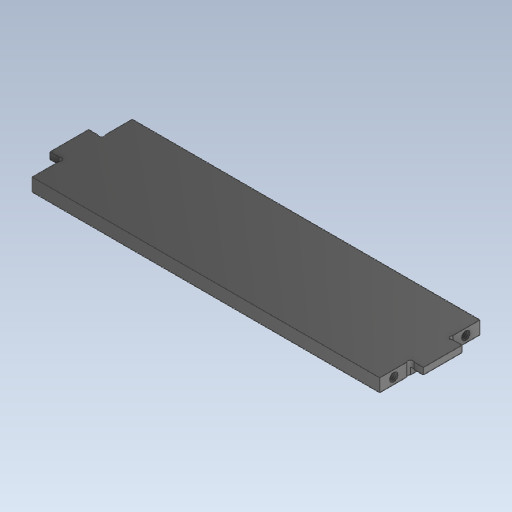
# Autodesk Inventor part: Cockpit_battery_bottom_frame
Saved by Autodesk Inventor 2020.4 (Build 244396000, 396)
## iProperties
Created: 2022-01-27
Part Number: Cockpit_battery_bottom_frame
Material: アセタール樹脂、黒
Document SubType Name: Modeling
Designer: Masato Kubotera
Density: 1.425 g/cm^3
Appearance: 滑らか - 黒
Author: Masato Kubotera
Autodesk Inventor part; units mm, degrees
ref_plane "YZ Plane" through (0, 0, 0) normal (1, 0, 0) x (0, 1, 0)
ref_plane "XZ Plane" through (0, 0, 0) normal (0, 1, 0) x (-1, 0, 0)
derived "Cockpit_side_frame_.ipt"
sketch "スケッチ2" plane through (0, 0, 0) normal (0, 1, 0) x (-1, 0, 0)
  line L0 (-28.5, -22.5) -> (86.5, -22.5) construction
  line L1 (86.5, -22.5) -> (86.5, -138.5)
  line L2 (86.5, -96) -> (-28.5, -96) construction
  line L3 (-28.5, -96) -> (-28.5, -22.5) construction
  line L4 (-28.5, -22.5) -> (86.5, -96) construction
  line L5 (86.5, -22.5) -> (-28.5, -96) construction
  line L6 (36.5, -101) -> (36.5, -133.5)
  line L7 (41.5, -138.5) -> (86.5, -138.5)
  arc A0 (62.6349, -70.4) -> (61.15, -71.8849) centre (61.8925, -71.1425) ccw
  arc A1 (71.15, -72.5349) -> (69.6651, -71.05) centre (70.4075, -71.7925) ccw
  line L8 (63.3349, -71.05) -> (69.6651, -71.05)
  line L9 (62.6349, -70.4) -> (70.3651, -70.4)
  line L10 (61.9, -71.1) -> (71.1, -71.1) construction
  arc A2 (63.3349, -71.05) -> (61.85, -72.5349) centre (62.5925, -71.7925) ccw
  line L11 (61.2, -70.45) -> (71.8, -70.45) construction
  line L12 (71.15, -72.5349) -> (71.15, -83.4651)
  line L13 (71.8, -78) -> (61.2, -78) construction
  line L14 (71.85, -71.8849) -> (71.85, -84.1151)
  line L15 (71.1, -71.1) -> (71.1, -84.9) construction
  line L16 (61.85, -72.5349) -> (61.85, -83.4651)
  line L17 (71.8, -70.45) -> (71.8, -85.55) construction
  line L18 (61.15, -71.8849) -> (61.15, -84.1151)
  line L19 (66.5, -70.45) -> (66.5, -85.55) construction
  line L20 (61.9, -84.9) -> (61.9, -71.1) construction
  line L21 (71.1, -71.1) -> (61.9, -84.9) construction
  line L22 (71.8, -70.45) -> (61.2, -85.55) construction
  line L23 (61.2, -70.45) -> (71.8, -85.55) construction
  line L24 (61.2, -85.55) -> (61.2, -70.45) construction
  line L25 (61.9, -71.1) -> (71.1, -84.9) construction
  arc A3 (71.85, -71.8849) -> (70.3651, -70.4) centre (71.1075, -71.1425) ccw
  line L26 (71.1, -84.9) -> (61.9, -84.9) construction
  line L27 (71.8, -85.55) -> (61.2, -85.55) construction
  arc A4 (61.85, -83.4651) -> (63.3349, -84.95) centre (62.5925, -84.2075) ccw
  arc A5 (61.15, -84.1151) -> (62.6349, -85.6) centre (61.8925, -84.8575) ccw
  line L28 (63.3349, -84.95) -> (69.6651, -84.95)
  line L29 (62.6349, -85.6) -> (70.3651, -85.6)
  arc A6 (69.6651, -84.95) -> (71.15, -83.4651) centre (70.4075, -84.2075) ccw
  arc A7 (70.3651, -85.6) -> (71.85, -84.1151) centre (71.1075, -84.8575) ccw
  line L30 (-23.5, -22.5) -> (-28.5, -27.5)
  line L31 (-28.5, -59.25) -> (86.5, -59.25) construction
  line L32 (29, -22.5) -> (29, -96) construction
  line L33 (-23.5, -96) -> (-28.5, -91)
  line L34 (-28.5, -27.5) -> (-28.5, -91)
  line L35 (-21, -25) -> (-26, -25) construction
  line L36 (-26, -25) -> (-26, -93.5) construction
  line L37 (-26, -93.5) -> (-21, -93.5) construction
  line L38 (-21, -93.5) -> (-21, -25) construction
  line L39 (-21, -25) -> (-26, -93.5) construction
  line L40 (-26, -25) -> (-21, -93.5) construction
  line L41 (-26.05, -46.7) -> (-20.95, -46.7)
  line L42 (-20.95, -46.7) -> (-20.95, -71.8)
  line L43 (-20.95, -71.8) -> (-26.05, -71.8)
  line L44 (-26.05, -71.8) -> (-26.05, -46.7)
  line L45 (-26.05, -46.7) -> (-20.95, -71.8) construction
  line L46 (-20.95, -46.7) -> (-26.05, -71.8) construction
  line L47 (-26, -46.75) -> (-21, -46.75) construction
  line L48 (-26, -71.75) -> (-21, -71.75) construction
  line L49 (-23.5, -25) -> (-23.5, -93.5) construction
  circle A8 centre (-23.5, -35) radius 3
  circle A9 centre (-23.5, -35) radius 1.6
  arc A10 (-24.5651, -46.7) -> (-26.05, -48.1849) centre (-25.3075, -47.4425) ccw
  arc A11 (-20.95, -48.1849) -> (-22.4349, -46.7) centre (-21.6925, -47.4425) ccw
  arc A12 (-22.4349, -71.8) -> (-20.95, -70.3151) centre (-21.6925, -71.0575) ccw
  arc A13 (-26.05, -70.3151) -> (-24.5651, -71.8) centre (-25.3075, -71.0575) ccw
  circle A14 centre (-23.5, -83.5) radius 1.6
  circle A15 centre (-23.5, -83.5) radius 3
  line L50 (31.5, -96) -> (36.5, -101)
  line L51 (-23.5, -96) -> (31.5, -96)
  line L52 (79, -67.5) -> (-21, -67.5) construction
  line L53 (-21, -67.5) -> (-21, -62.5) construction
  line L54 (-21, -62.5) -> (79, -62.5) construction
  line L55 (79, -62.5) -> (79, -67.5) construction
  line L56 (79, -67.5) -> (-21, -62.5) construction
  line L57 (-21, -67.5) -> (79, -62.5) construction
  line L58 (-21, -65) -> (79, -65) construction
  line L59 (29, -62.5) -> (29, -67.5) construction
  line L60 (4, -62.5) -> (4, -67.5) construction
  line L61 (54.05, -62.45) -> (3.95, -62.45)
  line L62 (3.95, -62.45) -> (3.95, -67.55)
  line L63 (3.95, -67.55) -> (54.05, -67.55)
  line L64 (54.05, -67.55) -> (54.05, -62.45)
  line L65 (54.05, -62.45) -> (3.95, -67.55) construction
  line L66 (3.95, -62.45) -> (54.05, -67.55) construction
  arc A16 (5.4349, -62.45) -> (3.95, -63.9349) centre (4.6925, -63.1925) ccw
  circle A17 centre (-3.5, -65) radius 3
  circle A18 centre (-3.5, -65) radius 1.6
  line L67 (54, -62.5) -> (54, -67.5) construction
  arc A19 (54.05, -63.9349) -> (52.5651, -62.45) centre (53.3075, -63.1925) ccw
  circle A20 centre (61.5, -65) radius 3
  circle A21 centre (61.5, -65) radius 1.6
  arc A22 (3.95, -66.0651) -> (5.4349, -67.55) centre (4.6925, -66.8075) ccw
  arc A23 (52.5651, -67.55) -> (54.05, -66.0651) centre (53.3075, -66.8075) ccw
  line L68 (-21, -88.5) -> (79, -88.5) construction
  line L69 (79, -88.5) -> (79, -93.5) construction
  line L70 (79, -93.5) -> (-21, -93.5) construction
  line L71 (-21, -93.5) -> (-21, -88.5) construction
  line L72 (-21, -88.5) -> (79, -93.5) construction
  line L73 (79, -88.5) -> (-21, -93.5) construction
  line L74 (-21, -91) -> (79, -91) construction
  line L75 (29, -88.5) -> (29, -93.5) construction
  line L76 (54.05, -91.05) -> (3.95, -91.05)
  line L77 (3.95, -91.05) -> (3.95, -88.45)
  line L78 (3.95, -88.45) -> (54.05, -88.45)
  line L79 (54.05, -88.45) -> (54.05, -91.05)
  line L80 (54.05, -91.05) -> (3.95, -88.45) construction
  line L81 (3.95, -91.05) -> (54.05, -88.45) construction
  line L82 (4, -88.5) -> (4, -91) construction
  line L83 (54, -88.5) -> (54, -91) construction
  line L84 (4, -89.75) -> (54, -89.75) construction
  arc A24 (6.05, -88.45) -> (3.95, -88.45) centre (5, -88.45) ccw
  arc A25 (54.05, -88.45) -> (51.95, -88.45) centre (53, -88.45) ccw
  arc A26 (51.95, -91.05) -> (54.05, -91.05) centre (53, -91.05) ccw
  arc A27 (3.95, -91.05) -> (6.05, -91.05) centre (5, -91.05) ccw
  circle A28 centre (-3.5, -91) radius 3
  circle A29 centre (-3.5, -91) radius 1.6
  circle A30 centre (61.5, -91) radius 3 construction
  circle A31 centre (61.5, -91) radius 1.6 construction
  line L85 (-23.5, -22.5) -> (64.25, -22.5)
  line L86 (64.25, -22.5) -> (64.25, -17.5)
  line L87 (64.25, -17.5) -> (72.25, -17.5)
  line L88 (72.25, -17.5) -> (72.25, -22.5)
  line L89 (72.25, -22.5) -> (79, -22.5)
  line L90 (79, -22.5) -> (79, -17.5)
  line L91 (86.5, -22.5) -> (86.5, -20)
  line L92 (79, -17.5) -> (84, -17.5)
  line L93 (84, -17.5) -> (86.5, -20)
  line L94 (68.25, -17.5) -> (68.25, -22.5) construction
  arc A32 (62.7651, -22.5) -> (64.25, -21.0151) centre (63.5075, -21.7575) ccw
  arc A33 (72.25, -21.0151) -> (73.7349, -22.5) centre (72.9925, -21.7575) ccw
  arc A34 (77.5151, -22.5) -> (79, -21.0151) centre (78.2575, -21.7575) ccw
  line L95 (-16, -88.5) -> (-16, -68.5) construction
  line L96 (-16, -68.5) -> (64, -68.5) construction
  line L97 (64, -68.5) -> (64, -88.5) construction
  line L98 (45.5, -86) -> (-16.5, -86)
  line L99 (-18.5, -84) -> (-18.5, -72)
  line L100 (-16.5, -70) -> (45.5, -70)
  line L101 (47.5, -72) -> (47.5, -84)
  line L102 (47.5, -86) -> (-18.5, -70) construction
  line L103 (-18.5, -86) -> (47.5, -70) construction
  arc A35 (-16.5, -70) -> (-18.5, -72) centre (-16.5, -72) ccw
  arc A36 (-18.5, -84) -> (-16.5, -86) centre (-16.5, -84) ccw
  arc A37 (45.5, -86) -> (47.5, -84) centre (45.5, -84) ccw
  arc A38 (47.5, -72) -> (45.5, -70) centre (45.5, -72) ccw
  line L104 (36.5, -133.5) -> (41.5, -138.5)
  line L105 (44, -131) -> (39, -131) construction
  line L106 (39, -131) -> (39, -96) construction
  line L107 (39, -96) -> (44, -96) construction
  line L108 (44, -96) -> (44, -131) construction
  line L109 (44, -131) -> (39, -96) construction
  line L110 (39, -131) -> (44, -96) construction
  line L111 (41.5, -96) -> (41.5, -131) construction
  line L112 (39, -113.5) -> (44, -113.5) construction
  line L113 (41.5, -107.5) -> (44, -107.5) construction
  line L114 (41.45, -107.45) -> (44.05, -107.45)
  line L115 (44.05, -107.45) -> (44.05, -119.55)
  line L116 (44.05, -119.55) -> (41.45, -119.55)
  line L117 (41.45, -119.55) -> (41.45, -107.45)
  line L118 (41.45, -107.45) -> (44.05, -119.55) construction
  line L119 (44.05, -107.45) -> (41.45, -119.55) construction
  arc A39 (44.05, -109.55) -> (44.05, -107.45) centre (44.05, -108.5) ccw
  arc A40 (42.9349, -107.45) -> (41.45, -108.9349) centre (42.1925, -108.1925) ccw
  arc A41 (44.05, -119.55) -> (44.05, -117.45) centre (44.05, -118.5) ccw
  line L120 (41.5, -119.5) -> (44, -119.5) construction
  arc A42 (41.45, -118.0651) -> (42.9349, -119.55) centre (42.1925, -118.8075) ccw
  line L121 (42.75, -107.5) -> (42.75, -119.5) construction
  circle A43 centre (41.5, -125.5) radius 3 construction
  circle A44 centre (41.5, -125.5) radius 1.6 construction
  circle A45 centre (41.5, -101.5) radius 3
  circle A46 centre (41.5, -101.5) radius 1.6
  circle A47 centre (-13.5, -55) radius 2
  line L122 (39, -131) -> (77.8645, -131) construction
  line L123 (77.8645, -131) -> (77.8645, -136) construction
  line L124 (77.8645, -136) -> (39, -136) construction
  line L125 (39, -136) -> (39, -131) construction
  line L126 (39, -131) -> (77.8645, -136) construction
  line L127 (77.8645, -131) -> (39, -136) construction
  line L128 (39, -133.5) -> (77.8645, -133.5) construction
  line L129 (58.4322, -131) -> (58.4322, -136) construction
  line L130 (58.4322, -133.5) -> (58.4322, -131) construction
  line L131 (50.8822, -130.95) -> (65.9822, -130.95)
  line L132 (65.9822, -130.95) -> (65.9822, -133.55)
  line L133 (65.9822, -133.55) -> (50.8822, -133.55)
  line L134 (50.8822, -133.55) -> (50.8822, -130.95)
  line L135 (50.8822, -130.95) -> (65.9822, -133.55) construction
  line L136 (65.9822, -130.95) -> (50.8822, -133.55) construction
  line L137 (50.9322, -131) -> (50.9322, -133.5) construction
  arc A48 (52.9822, -130.95) -> (50.8822, -130.95) centre (51.9322, -130.95) ccw
  arc A49 (50.8822, -132.0651) -> (52.3672, -133.55) centre (51.6247, -132.8075) ccw
  arc A50 (65.9822, -130.95) -> (63.8822, -130.95) centre (64.9322, -130.95) ccw
  arc A51 (64.4973, -133.55) -> (65.9822, -132.0651) centre (65.2398, -132.8075) ccw
  line L138 (65.9322, -131) -> (65.9322, -133.5) construction
  line L139 (50.9322, -132.25) -> (65.9322, -132.25) construction
  circle A52 centre (72.4322, -133.5) radius 1.6 construction
  circle A53 centre (72.4322, -133.5) radius 3 construction
  circle A54 centre (44.4322, -133.5) radius 3
  circle A55 centre (44.4322, -133.5) radius 1.6
  line L140 (48.5, -96) -> (77, -96)
  line L141 (79, -98) -> (79, -126.5)
  line L142 (77, -128.5) -> (48.5, -128.5)
  line L143 (46.5, -126.5) -> (46.5, -98)
  line L144 (46.5, -96) -> (79, -128.5) construction
  line L145 (79, -96) -> (46.5, -128.5) construction
  arc A56 (48.5, -96) -> (46.5, -98) centre (48.5, -98) ccw
  arc A57 (46.5, -126.5) -> (48.5, -128.5) centre (48.5, -126.5) ccw
  arc A58 (77, -128.5) -> (79, -126.5) centre (77, -126.5) ccw
  arc A59 (79, -98) -> (77, -96) centre (77, -98) ccw
  line L146 (79, -91.1738) -> (84, -91.1738) construction
  line L147 (84, -91.1738) -> (84, -136) construction
  line L148 (84, -136) -> (79, -136) construction
  line L149 (79, -136) -> (79, -91.1738) construction
  line L150 (79, -91.1738) -> (84, -136) construction
  line L151 (84, -91.1738) -> (79, -136) construction
  line L152 (81.5, -91.1738) -> (81.5, -136) construction
  circle A60 centre (81.5, -93.6738) radius 1.475
  circle A61 centre (81.5, -98.6738) radius 1.475
  circle A62 centre (81.5, -103.6738) radius 1.475
  circle A63 centre (81.5, -133.5) radius 1.6
  arc A64 (84, -91.1738) -> (79, -91.1738) centre (81.5, -133.5) ccw construction
  arc A65 (84.0111, -91.0742) -> (78.9889, -91.0742) centre (81.5, -133.5) ccw construction
  line L153 (86.5, -133.5) -> (81.5, -138.5)
  arc A66 (79, -131) -> (84, -136) centre (81.5, -133.5) ccw construction
  line L154 (79, -65) -> (84, -65) construction
  line L155 (84, -65) -> (84, -91) construction
  line L156 (84, -91) -> (79, -91) construction
  line L157 (79, -91) -> (79, -65) construction
  line L158 (79, -65) -> (84, -91) construction
  line L159 (84, -65) -> (79, -91) construction
  line L160 (79, -78) -> (84, -78) construction
  line L161 (81.5, -65) -> (81.5, -91) construction
  line L162 (79, -73) -> (84, -73) construction
  line L163 (78.95, -72.95) -> (86.5, -72.95)
  line L164 (84.05, -72.95) -> (84.05, -83.05) construction
  line L165 (84.05, -83.05) -> (78.95, -83.05)
  line L166 (78.95, -83.05) -> (78.95, -72.95)
  line L167 (78.95, -72.95) -> (84.05, -83.05) construction
  line L168 (84.05, -72.95) -> (78.95, -83.05) construction
  arc A67 (80.4349, -72.95) -> (78.95, -74.4349) centre (79.6925, -73.6925) ccw
  arc A68 (78.95, -81.5651) -> (80.4349, -83.05) centre (79.6925, -82.3075) ccw
  line L169 (79, -83) -> (84, -83) construction
  circle A69 centre (81.5, -68) radius 1.6
  circle A70 centre (81.5, -68) radius 3
  circle A71 centre (81.5, -88) radius 1.6
  circle A72 centre (81.5, -88) radius 3
  line L170 (84.05, -83.05) -> (86.5, -83.05)
  circle A73 centre (81.5, -133.5) radius 3
  line L171 (75.625, -22.5) -> (75.625, -27.147) construction
  line L172 (60.875, -22.5) -> (60.875, -27.147) construction
  line L173 (64.25, -22.5) -> (72.25, -22.5)
  point P0 (0, 0)
  point P1 (29, -59.25)
  point P2 (-25.7227, -96)
  point P3 (61.85, -71.05)
  point P4 (61.15, -70.4)
  point P5 (66.5, -78)
  point P6 (-23.5, -59.25)
  point P7 (29, -65)
  point P8 (29, -91)
  point P9 (29, -89.75)
  point P10 (29, -89.75)
  point P11 (52.5, -22)
  point P12 (14.5, -78)
  point P13 (-18.5, -61)
  point P14 (47.5, -61)
  point P15 (41.5, -113.5)
  point P16 (42.75, -113.5)
  point P17 (58.4322, -133.5)
  point P18 (58.4322, -132.25)
  point P19 (62.75, -112.25)
  point P20 (81.5, -113.5869)
  point P21 (81.5, -78)
  dimension "d1" = 131
  dimension "d2" = 5
  dimension "d9" = 2.5
  measures "d1" vertical distance of L122.start point (0, 0)
  measures "d2" distance of L124.end L122.start
  measures "d9" distance of L137.start L137.end
ref_plane "作業平面1" through (0, 0, -131) normal (0, 0, 1) x (1, 0, 0)
sketch "スケッチ3" plane through (0, 0, -131) normal (0, 0, 1) x (1, 0, 0)
  line L0 (-77.8645, -135) -> (-39, -135)
  line L1 (-39, -135) -> (-39, 0)
  line L2 (-39, 0) -> (-77.8645, 0)
  line L3 (-77.8645, 0) -> (-77.8645, -135)
  line L4 (-77.8645, -135) -> (-39, 0) construction
  line L5 (-39, -135) -> (-77.8645, 0) construction
  line L6 (-65.9322, 0) -> (-65.9322, 5)
  line L7 (-65.9322, 5) -> (-50.9322, 5)
  line L8 (-50.9322, 5) -> (-50.9322, 0)
  line L9 (-58.4322, 0) -> (-58.4322, -135) construction
  arc A0 (-67.4172, 0) -> (-65.9322, 1.4849) centre (-66.6747, 0.7425) ccw
  line L10 (-58.4322, 5) -> (-58.4322, 0) construction
  arc A1 (-50.9322, 1.4849) -> (-49.4473, 0) centre (-50.1898, 0.7425) ccw
  line L11 (-77.8645, -67.5) -> (-39, -67.5)
  line L12 (-45.3645, -15) -> (-43.5, -15)
  line L13 (-41.5, -13) -> (-41.5, -7)
  line L14 (-43.5, -5) -> (-45.3645, -5)
  line L15 (-47.3645, -7) -> (-47.3645, -13)
  line L16 (-47.3645, -15) -> (-41.5, -5) construction
  line L17 (-41.5, -15) -> (-47.3645, -5) construction
  line L18 (-51.8645, -5) -> (-65, -5)
  line L19 (-49.8645, -7) -> (-49.8645, -16.0799)
  line L20 (-49.8932, -16.4177) -> (-56.461, -54.746)
  line L21 (-43.5, -17.5) -> (-45.678, -17.5)
  line L22 (-47.6493, -19.1622) -> (-55.8744, -67.1622)
  line L23 (-41.5, -19.5) -> (-41.5, -67.5)
  line L24 (-44.4322, -5) -> (-44.4322, 0) construction
  line L25 (-71.5, -15) -> (-73.3645, -15)
  line L26 (-75.3645, -13) -> (-75.3645, -7)
  line L27 (-73.3645, -5) -> (-71.5, -5)
  line L28 (-69.5, -7) -> (-69.5, -13)
  line L29 (-67, -7) -> (-67, -16.0799)
  line L30 (-66.9713, -16.4177) -> (-60.4035, -54.746)
  line L31 (-73.3645, -17.5) -> (-71.1864, -17.5)
  line L32 (-69.2152, -19.1622) -> (-60.9901, -67.1622)
  line L33 (-75.3645, -19.5) -> (-75.3645, -67.5)
  line L34 (-45.3645, -120) -> (-43.5, -120)
  line L35 (-41.5, -122) -> (-41.5, -128)
  line L36 (-43.5, -130) -> (-45.3645, -130)
  line L37 (-47.3645, -128) -> (-47.3645, -122)
  line L38 (-51.8645, -130) -> (-65, -130)
  line L39 (-49.8645, -128) -> (-49.8645, -118.9201)
  line L40 (-49.8932, -118.5823) -> (-56.461, -80.254)
  line L41 (-43.5, -117.5) -> (-45.678, -117.5)
  line L42 (-47.6493, -115.8378) -> (-55.8744, -67.8378)
  line L43 (-41.5, -115.5) -> (-41.5, -67.5)
  line L44 (-69.2152, -115.8378) -> (-60.9901, -67.8378)
  line L45 (-73.3645, -117.5) -> (-71.1864, -117.5)
  line L46 (-71.5, -120) -> (-73.3645, -120)
  line L47 (-69.5, -128) -> (-69.5, -122)
  line L48 (-73.3645, -130) -> (-71.5, -130)
  line L49 (-75.3645, -122) -> (-75.3645, -128)
  line L50 (-75.3645, -115.5) -> (-75.3645, -67.5)
  line L51 (-67, -128) -> (-67, -118.9201)
  line L52 (-66.9713, -118.5823) -> (-60.4035, -80.254)
  arc A2 (-73.3645, -5) -> (-75.3645, -7) centre (-73.3645, -7) ccw
  arc A3 (-69.5, -7) -> (-71.5, -5) centre (-71.5, -7) ccw
  arc A4 (-71.5, -15) -> (-69.5, -13) centre (-71.5, -13) ccw
  arc A5 (-75.3645, -13) -> (-73.3645, -15) centre (-73.3645, -13) ccw
  arc A6 (-65, -5) -> (-67, -7) centre (-65, -7) ccw
  arc A7 (-49.8645, -7) -> (-51.8645, -5) centre (-51.8645, -7) ccw
  arc A8 (-45.3645, -5) -> (-47.3645, -7) centre (-45.3645, -7) ccw
  arc A9 (-41.5, -7) -> (-43.5, -5) centre (-43.5, -7) ccw
  arc A10 (-47.3645, -13) -> (-45.3645, -15) centre (-45.3645, -13) ccw
  arc A11 (-43.5, -15) -> (-41.5, -13) centre (-43.5, -13) ccw
  arc A12 (-41.5, -19.5) -> (-43.5, -17.5) centre (-43.5, -19.5) ccw
  arc A13 (-45.678, -17.5) -> (-47.6493, -19.1622) centre (-45.678, -19.5) ccw
  arc A14 (-49.8932, -16.4177) -> (-49.8645, -16.0799) centre (-51.8645, -16.0799) ccw
  arc A15 (-67, -16.0799) -> (-66.9713, -16.4177) centre (-65, -16.0799) ccw
  arc A16 (-73.3645, -17.5) -> (-75.3645, -19.5) centre (-73.3645, -19.5) ccw
  arc A17 (-69.2152, -19.1622) -> (-71.1864, -17.5) centre (-71.1864, -19.5) ccw
  arc A18 (-60.9901, -67.8378) -> (-60.9901, -67.1622) centre (-62.9614, -67.5) ccw
  arc A19 (-55.8744, -67.1622) -> (-55.8744, -67.8378) centre (-53.9031, -67.5) ccw
  arc A20 (-60.4035, -54.746) -> (-56.461, -54.746) centre (-58.4322, -54.4082) ccw
  arc A21 (-56.461, -80.254) -> (-60.4035, -80.254) centre (-58.4322, -80.5918) ccw
  arc A22 (-75.3645, -115.5) -> (-73.3645, -117.5) centre (-73.3645, -115.5) ccw
  arc A23 (-71.1864, -117.5) -> (-69.2152, -115.8378) centre (-71.1864, -115.5) ccw
  arc A24 (-73.3645, -120) -> (-75.3645, -122) centre (-73.3645, -122) ccw
  arc A25 (-69.5, -122) -> (-71.5, -120) centre (-71.5, -122) ccw
  arc A26 (-75.3645, -128) -> (-73.3645, -130) centre (-73.3645, -128) ccw
  arc A27 (-71.5, -130) -> (-69.5, -128) centre (-71.5, -128) ccw
  arc A28 (-67, -128) -> (-65, -130) centre (-65, -128) ccw
  arc A29 (-66.9713, -118.5823) -> (-67, -118.9201) centre (-65, -118.9201) ccw
  arc A30 (-49.8645, -118.9201) -> (-49.8932, -118.5823) centre (-51.8645, -118.9201) ccw
  arc A31 (-51.8645, -130) -> (-49.8645, -128) centre (-51.8645, -128) ccw
  arc A32 (-47.3645, -128) -> (-45.3645, -130) centre (-45.3645, -128) ccw
  arc A33 (-45.3645, -120) -> (-47.3645, -122) centre (-45.3645, -122) ccw
  arc A34 (-41.5, -122) -> (-43.5, -120) centre (-43.5, -122) ccw
  arc A35 (-43.5, -130) -> (-41.5, -128) centre (-43.5, -128) ccw
  arc A36 (-47.6493, -115.8378) -> (-45.678, -117.5) centre (-45.678, -115.5) ccw
  arc A37 (-43.5, -117.5) -> (-41.5, -115.5) centre (-43.5, -115.5) ccw
  line L53 (-42.8322, 0) -> (-46.0322, 0) projected
  point P0 (0, 0)
  point P1 (-58.4322, -67.5)
  point P2 (-49.4473, 0)
  point P3 (-50.9322, 0)
  point P4 (-50.9322, 1.4849)
  point P5 (-44.4322, -10)
  point P6 (-49.8645, -5)
  point P7 (-67, -5)
  point P8 (-49.8645, -16.25)
  point P9 (-58.4322, -66.25)
  point P10 (-41.5, -17.5)
  point P11 (-47.3645, -17.5)
  point P12 (-55.9322, -67.5)
  point P13 (-69.5, -15)
  point P14 (-75.3645, -5)
  point P15 (-75.3645, -15)
  point P16 (-69.5, -5)
  point P17 (-67, -16.25)
  point P18 (-75.3645, -17.5)
  point P19 (-69.5, -17.5)
  point P20 (-60.9322, -67.5)
  point P21 (-47.3645, -120)
  point P22 (-41.5, -130)
  point P23 (-41.5, -120)
  point P24 (-47.3645, -130)
  point P25 (-49.8645, -130)
  point P26 (-67, -130)
  point P27 (-49.8645, -118.75)
  point P28 (-58.4322, -68.75)
  point P29 (-41.5, -117.5)
  point P30 (-47.3645, -117.5)
  point P31 (-69.5, -117.5)
  point P32 (-75.3645, -117.5)
  point P33 (-69.5, -120)
  point P34 (-75.3645, -120)
  point P35 (-69.5, -130)
  point P36 (-75.3645, -130)
  point P37 (-67, -118.75)
  point P38 (-60.9614, -67.5)
  point P39 (-55.9031, -67.5)
  dimension "d4" = 1.05
  dimension "d5" = 5
  dimension "d6" = 135
  dimension "d24" = 2.5
  dimension "d25" = 5
  dimension "d26" = 2.5
  dimension "d30" = 10
  dimension "d31" = 11.25
  dimension "d32" = 2.5
  dimension "d33" = 5
  dimension "d34" = 2
  constraints: 104 end point, 78 point on line, 77 point on circle, 72 tangent, 38 centre point, 35 equal radius, 30 symmetric about line, 9 midpoint, 6 perpendicular, 4 horizontal, 4 parallel, 4 vertical, 2 coincident, 2 collinear, 7 other
  measures "d4" radius of A0
  measures "d5" distance of L6.start L6.end
  measures "d6" distance of L3.start L0.start
  measures "d24" horizontal distance of L1.end L16.end
  measures "d25" vertical distance of L1.end L16.end
  measures "d26" distance of point (-41.5, -17.5) L17.start
  measures "d30" distance of L17.start L16.end
  measures "d31" distance of point (-49.864, -5) point (-49.864, -16.25)
  measures "d32" distance of point (-49.864, -5) L17.end
  measures "d33" distance of point (-55.932, -67.5) point (-60.932, -67.5)
  measures "d34" radius of A2
extrude "押し出し1" add sketch "スケッチ3" against normal blind 5 contours L3 L2 A0 A1 L1 L11 L23 A12 L21 A13 L22 A19 A18 L32 A17 L31 A16 L33
extrude "押し出し2" add sketch "スケッチ3" against normal blind 2.5 contours A0 L6 L7 L8 A1 L2
hole "穴1" at (-72.4322, 0, -133.5) at (-44.4322, 0, -133.5) direction (0, -1, 0) diameter 3.242 depth 5 tip angle 118 thread size "M4x0.7" class "6H" standard "ISO Metric profile"
extrude "押し出し3" add sketch "スケッチ3" against normal blind 0.5 contours L33 A16 L31 A17 L32 A18 L11 | L11 A19 L22 A13 L21 A12 L23 | A10 L15 A8 L14 A9 L13 A11 L12 | A7 L19 A14 L20 A20 L30 A15 L29 A6 L18 | L25 A5 L26 A2 L27 A3 L28 A4
mirror "ミラー1" about plane through (-75.3645, -67.5, -131) normal (0, -1, 0)
equation "\"d26\" = d24"
equation "\"d32\" = d24"
equation "\"d7\" = d2"
equation "\"d10\" = d9"
equation "\"d3\" = -d1"
